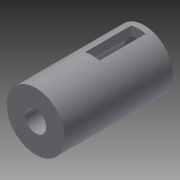
# Autodesk Inventor part: axe
Saved by Autodesk Inventor 2014 SP1 (Build 180222100, 222)
## iProperties
Created: 2015-01-28
Part Number: axe
Material: Générique
Document SubType Name: Modeling
Designer: astralien3000
Density: 1 g/cm^3
Appearance: Par défaut
Author: astralien3000
Autodesk Inventor part; units mm, degrees
ref_plane "YZ Plane" through (0, 0, 0) normal (1, 0, 0) x (0, 1, 0)
ref_plane "XZ Plane" through (0, 0, 0) normal (0, 1, 0) x (-1, 0, 0)
ref_plane "XY Plane" through (0, 0, 0) normal (0, 0, 1) x (1, 0, 0)
sketch "Esquisse1" plane through (0, 0, 0) normal (0, 1, 0) x (-1, 0, 0)
  circle A0 centre (0, 0) radius 1.45
  circle A1 centre (0, 0) radius 4
  dimension "d0" = 8
  dimension "d1" = 2.9
  constraints: 2 centre point, 2 coincident
  measures "d0" diameter of A1
  measures "d1" diameter of A0
extrude "Extrusion1" add sketch "Esquisse1" along normal blind 7
sketch "Esquisse2" plane through (0, 7, 0) normal (0, 1, 0) x (1, 0, 0)
  circle A0 centre (0, 0) radius 1.45 projected
  circle A1 centre (0, 0) radius 4 projected
  arc A2 (-2.3049, 1.5) -> (2.3049, 1.5) centre (0, 0) ccw
  line L0 (-2.3049, 1.5) -> (2.3049, 1.5)
  arc A3 (2.3049, 1.5) -> (-2.3049, 1.5) centre (0, 0) ccw construction
  dimension "d4" = 5.5
  dimension "d5" = 1.5
  constraints: 4 point on circle, 2 centre point, 2 end point, 1 coincident, 1 horizontal
  measures "d4" diameter of A2
  measures "d5" distance from line of A0.centre L0
extrude "Extrusion2" add sketch "Esquisse2" along normal blind 8 contours A1
sketch "Esquisse3" plane through (-2.3049, 7, -1.5) normal (0, 0, 1) x (1, 0, 0)
  line L0 (4.6098, 0) -> (0, 0) projected
  line L1 (4.6098, 0) -> (4.6098, 8) projected
  line L2 (0, 8) -> (4.6098, 8) projected
  line L3 (1.3049, 7.2) -> (3.3049, 7.2)
  line L4 (3.3049, 7.2) -> (3.3049, 0.8)
  line L5 (3.3049, 0.8) -> (1.3049, 0.8)
  line L6 (1.3049, 0.8) -> (1.3049, 7.2)
  point P0 (2.3049, -7)
  dimension "d8" = 2
  dimension "d9" = 0.8
  dimension "d10" = 0.8
  dimension "d11" = 1.3049
  dimension "d12" = 4.6098
  constraints: 8 end point, 2 parallel, 1 horizontal, 1 perpendicular
  measures "d8" distance between parallel lines of L6 L4
  measures "d9" distance between parallel lines of L5 L0
  measures "d10" distance between parallel lines of L2 L3
  measures "d11" distance between parallel lines of L1 L4
  measures "d12" distance of L2.start L1.end
extrude "Extrusion3" cut sketch "Esquisse3" along normal through all both and the other way through all
equation "\"d9\" = d10"
equation "\"d11\" = -0.5 * d8 + 0.5 * d12"
